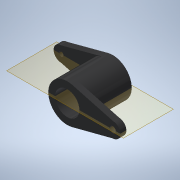
# Autodesk Inventor part: steering_stand_off
Saved by Autodesk Inventor 2020 (Build 240168000, 168)
## iProperties
Created: 2015-12-07
Part Number: steering_stand_off
Material: Goma
Document SubType Name: Modeling
Designer: MIGUEL ANGEL
Density: 0.93 g/cm^3
Appearance: Goma - Negro - Versión 1.1
Author: MIGUEL ANGEL
Autodesk Inventor part; units mm, degrees
ref_plane "YZ Plane" through (0, 0, 0) normal (1, 0, 0) x (0, 1, 0)
ref_plane "XZ Plane" through (0, 0, 0) normal (0, 1, 0) x (-1, 0, 0)
sketch "Boceto1" plane through (0, 0, 0) normal (0, 1, 0) x (-1, 0, 0)
  circle A0 centre (0, 0) radius 12.5
  dimension "d0" = 25
  constraints: 1 centre point, 1 coincident
  measures "d0" diameter of A0
extrude "Extrusión1" add sketch "Boceto1" along normal blind 30
sketch "Boceto2" plane through (0, 0, 0) normal (0, -1, 0) x (1, 0, 0)
  circle A0 centre (0, 0) radius 8
  dimension "d3" = 16
  constraints: 1 centre point, 1 coincident
  measures "d3" diameter of A0
extrude "Extrusión2" cut sketch "Boceto2" against normal through all
sketch "Boceto3" plane through (0, 30, 0) normal (0, 1, 0) x (1, 0, 0)
  line L0 (6, 10.3923) -> (12, 0)
  line L1 (12, 0) -> (6, -10.3923)
  line L2 (6, -10.3923) -> (-6, -10.3923)
  line L3 (-6, -10.3923) -> (-12, 0)
  line L4 (-12, 0) -> (-6, 10.3923)
  line L5 (-6, 10.3923) -> (6, 10.3923)
  point P0 (0, 0)
  point P1 (0, 0)
  point P2 (0, 10.3923)
  dimension "d6" = 12
  constraints: 12 end point, 1 coincident, 1 midpoint, 1 vertical alignment, 13 other
  measures "d6" distance of L4.end L0.start
extrude "Extrusión3" cut sketch "Boceto3" against normal blind 4
sketch "Boceto4" plane through (0, 0, 0) normal (0, -1, 0) x (1, 0, 0)
  circle A0 centre (0, 0) radius 12.5 projected
  arc A1 (30.0364, -5.1409) -> (30.0797, 4.8584) centre (29.9997, -0.141) ccw
  line L0 (30.0364, -5.1409) -> (3.1308, -12.1016)
  circle A2 centre (0, 0) radius 12.5 projected
  line L1 (30.0797, 4.8584) -> (3.2448, 12.0715)
  dimension "d9" = 10
  dimension "d10" = 30
  constraints: 6 point on circle, 4 end point, 2 tangent, 1 centre point
  measures "d9" diameter of A1
  measures "d10" distance of point (0, 0) A1.centre
extrude "Extrusión4" add sketch "Boceto4" against normal blind 4 contours A0 L1 A1 L0
sketch "Boceto5" plane through (0, 30, 0) normal (0, 1, 0) x (1, 0, 0)
  arc A0 (-30, 5) -> (-30, -5) centre (-30, 0) ccw
  line L0 (-30, -5) -> (-3.1942, -12.085)
  circle A1 centre (0, 0) radius 12.5 projected
  line L1 (-30, 5) -> (-3.1942, 12.085)
  dimension "d13" = 10
  dimension "d14" = 30
  constraints: 4 end point, 4 point on circle, 2 tangent, 1 centre point
  measures "d13" diameter of A0
  measures "d14" distance of A0.centre point (0, 0)
extrude "Extrusión5" add sketch "Boceto5" against normal blind 4 contours L1 A1 L0 A0
hole "Agujero1" at (29.9997, 4, -0.141) direction (0, -1, 0) diameter 4 depth 8 tip angle 118
hole "Agujero2" at (-30, 30, 0) direction (0, -1, 0) diameter 3 depth 8 tip angle 118
